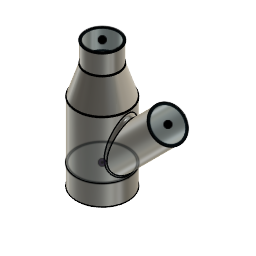
2.25 2 in 4 out pipe V3 (Autodesk Fusion 360 design; units mm, degrees)
Autodesk Fusion 360 part; units mm, degrees
sketch "Sketch1" plane through (0, 0, 0) normal (0, 0, 1) x (1, 0, 0)
  circle A0 centre (0, 0) radius 47
  circle A1 centre (0, 0) radius 49.5
  dimension "d1" = 94
  dimension "d2" = 2.5
  constraint coincident A0.centre A1.centre
  measures "d1" diameter of A0
ref_plane "WorkPlane1" through (0, 0, 203.2) normal (0, 0, 1) x (1, 0, 0)
sketch "Sketch2" plane through (0, 0, 203.2) normal (0, 0, 1) x (1, 0, 0)
  circle A0 centre (0, 0) radius 28.95
  circle A1 centre (0, 0) radius 31.45
  dimension "d4" = 57.9
  dimension "d5" = 2.5
  constraint coincident A0.centre A1.centre
  measures "d4" diameter of A0
ref_plane "WorkPlane2" through (0, 12.125, 0) normal (0.707107, 0, 0.707107) x (0, 1, 0)
ref_plane "WorkPlane3" through (125.7236, 12.125, 125.7236) normal (0.707107, 0, 0.707107) x (0, 1, 0)
sketch "Sketch3" plane through (125.7236, 0, 125.7236) normal (0.707107, 0, 0.707107) x (0, 1, 0)
  circle A0 centre (0, 0) radius 28.95
  circle A1 centre (0, 0) radius 31.45
  dimension "d10" = 57.9
  dimension "d11" = 2.5
  constraint coincident A0.centre A1.centre
  measures "d10" diameter of A0
extrude "Extrude1" add sketch "Sketch1" along normal blind 110 makes body 1
extrude "Extrude2" add sketch "Sketch2" against normal blind 38.1 separate body makes body 2
extrude "Extrude3" add sketch "Sketch3" against normal blind 180 separate body makes body 3
sketch "Sketch4" plane through (0, 0, 0) normal (0, 1, 0) x (1, 0, 0)
  line L0 (-49.5, -110) -> (49.5, -110)
  line L1 (-49.5, 0) -> (49.5, 0)
  line L2 (31.45, -165.1) -> (-31.45, -165.1)
  line L3 (-31.45, -203.2) -> (31.45, -203.2)
  line L4 (20.6829, 23.7941) -> (-23.7941, -20.6829)
  line L5 (103.4851, -147.9621) -> (147.9621, -103.4851)
  line L6 (-1.5556, 1.5556) -> (125.7236, -125.7236) construction
  line L7 (-1.5556, 1.5556) -> (-102.9075, 102.9075)
  line L8 (-1.5556, 1.5556) -> (136.8577, 1.5556) construction
  line L9 (0, -203.2) -> (0, -165.1)
  line L10 (0, -165.1) -> (0, -110)
  line L11 (47, -110) -> (-47, -110)
  line L12 (47, 0) -> (-47, 0)
  line L13 (-102.9075, 102.9075) -> (125.7236, -125.7236)
  line L14 (-31.45, -165.1) -> (-49.5, -110)
  line L15 (-47, -110) -> (-28.95, -165.1)
  line L16 (31.45, -165.1) -> (49.5, -110)
  line L17 (47, -110) -> (28.95, -165.1)
  dimension "d18" = 135
  constraint midpoint L4 L6.start
  constraint midpoint L5 L6.end
  constraint horizontal L8
  constraint midpoint L3 L9.start
  constraint midpoint L2 L9.end
  constraint midpoint L0 L10.end
  constraint coincident L2.end L14.start
  constraint coincident L0.start L14.end
  constraint coincident L11.end L15.start
  constraint coincident L2 L15.end
  constraint parallel L14 L15
  constraint coincident L2.start L16.start
  constraint coincident L0.end L16.end
  constraint coincident L11.start L17.start
  constraint coincident L2 L17.end
  constraint parallel L16 L17
  measures "d18" angle of L7 L8
extrude "Extrude4" cut sketch "Sketch1" along normal mid plane 200 contours A0 bodies 3
extrude "Extrude5" add sketch "Sketch1" against normal blind 40 bodies 1
extrude "Extrude7" cut sketch "Sketch3" against normal blind 190 contours A0 bodies 1
revolve "Revolve1" add sketch "Sketch4" angle 360 about axis through (0, 0, 165.1) along (0, 0, -1) contours L0 L2 L14 L15 bodies 1 2
combine "Combine1" operation add target body 1 tool bodies 3
fillet "Fillet1" radius 5 1 edges at (39.6986, 29.5683, 54.8537) on bodies 1
fillet "Fillet2" radius 5 1 edges at (38.2393, 27.3271, 51.7558) on bodies 1
fillet "Fillet3" radius 5 1 edges at (-46.1502, -17.9, 110) on bodies 1
fillet "Fillet4" radius 5 1 edges at (-29.3217, 11.3728, 165.1) on bodies 1
fillet "Fillet5" radius 5 1 edges at (-43.8194, 16.9959, 110) on bodies 1
fillet "Fillet6" radius 5 1 edges at (-26.9909, -10.4688, 165.1) on bodies 1
fillet "Fillet7" radius 1 3 faces at (30.3918, -3.0007, 203.2) (145.3956, -12.5972, 106.0516) (48.3074, -4.7942, -40) on bodies 1 2
equation "d1 = fourInHose"
equation "d2 = wallThickness"
equation "d4 = smallConnector"
equation "d5 = wallThickness"
equation "wallThickness = 2.5 mm"
equation "smallConnector = 57.9 mm"
equation "d10 = smallConnector"
equation "d11 = wallThickness"
equation "fourInHose = 94 mm"
